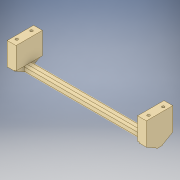
# Autodesk Inventor part: Handle
Saved by Autodesk Inventor 2019 (Build 230136000, 136)
## iProperties
Created: 2020-03-14
Part Number: Handle
Material: Generic
Document SubType Name: Modeling
Designer: james
Density: 1 g/cm^3
Appearance: Beige
Author: james
Autodesk Inventor part; units mm, degrees
ref_plane "YZ Plane" through (0, 0, 0) normal (1, 0, 0) x (0, 1, 0)
ref_plane "XZ Plane" through (0, 0, 0) normal (0, 1, 0) x (-1, 0, 0)
ref_plane "XY Plane" through (0, 0, 0) normal (0, 0, 1) x (1, 0, 0)
sketch "Sketch1" plane through (0, 0, 0) normal (1, 0, 0) x (0, 1, 0)
  line L0 (7.7549, 10.0308) -> (1.4049, 10.0308)
  line L1 (-1.7701, 6.8558) -> (-1.7701, 0.5058)
  line L2 (1.4049, -2.6692) -> (7.7549, -2.6692)
  line L3 (10.9299, 0.5058) -> (10.9299, 6.8558)
  arc A0 (10.9299, 6.8558) -> (7.7549, 10.0308) centre (7.7549, 6.8558) ccw
  arc A1 (7.7549, -2.6692) -> (10.9299, 0.5058) centre (7.7549, 0.5058) ccw
  arc A2 (-1.7701, 0.5058) -> (1.4049, -2.6692) centre (1.4049, 0.5058) ccw
  arc A3 (1.4049, 10.0308) -> (-1.7701, 6.8558) centre (1.4049, 6.8558) ccw
  point P0 (0, 0)
  point P1 (10.9299, 10.0308)
  point P2 (-1.7701, -2.6692)
  point P3 (-1.7701, 10.0308)
  dimension "d0" = 12.7
  dimension "d1" = 12.7
  dimension "d2" = 3.175
  constraints: 8 end point, 8 point on circle, 8 tangent, 6 point on line, 4 centre point, 3 equal radius, 2 parallel, 1 horizontal, 1 perpendicular
  measures "d0" distance of point (-1.77, 10.031) point (-1.77, -2.669)
  measures "d1" distance of point (10.93, 10.031) point (-1.77, 10.031)
  measures "d2" radius of A0
extrude "Extrusion1" add sketch "Sketch1" along normal blind 241.3
sketch "Sketch2" plane through (0, 10.9299, 6.8558) normal (0, 1, 0) x (1, 0, 0)
  line L0 (0, -22.225) -> (15.24, -22.225)
  line L1 (15.24, -22.225) -> (15.24, 28.575)
  line L2 (15.24, 28.575) -> (0, 28.575)
  line L3 (0, 28.575) -> (0, -22.225)
  line L4 (0, -3.175) -> (241.3, -3.175) projected
  line L5 (0, 9.525) -> (241.3, 9.525) projected
  line L6 (226.06, -22.225) -> (241.3, -22.225)
  line L7 (241.3, -22.225) -> (241.3, 28.575)
  line L8 (241.3, 28.575) -> (226.06, 28.575)
  line L9 (226.06, 28.575) -> (226.06, -22.225)
  line L10 (241.3, 6.35) -> (241.3, 0) projected
  point P0 (0, 6.8558)
  dimension "d5" = 19.05
  dimension "d6" = 19.05
  dimension "d7" = 15.24
  dimension "d8" = 0
  dimension "d9" = 19.05
  dimension "d10" = 19.05
  dimension "d11" = 15.24
  constraints: 16 end point, 4 parallel, 2 horizontal, 2 perpendicular
  measures "d5" distance between parallel lines of L4 L0
  measures "d6" distance between parallel lines of L5 L2
  measures "d7" distance between parallel lines of L1 L3
  measures "d8" distance between parallel lines of L10 L7
  measures "d9" distance between parallel lines of L5 L8
  measures "d10" distance between parallel lines of L4 L6
  measures "d11" distance between parallel lines of L7 L9
extrude "Extrusion2" add sketch "Sketch2" along normal blind 38.1 contours L3 L4 L1 L0 | L3 L5 L1 L4 | L3 L2 L1 L5 | L9 L5 L7 L4 | L4 L7 L6 L9 | L9 L8 L7 L5
sketch "Sketch4" plane through (241.3, 0, 0) normal (1, 0, 0) x (0, 0, -1)
  line L0 (-29.0808, 10.9299) -> (-6.8558, 10.9299) projected
  line L1 (-0.5058, 10.9299) -> (21.7192, 10.9299) projected
  line L2 (-6.8558, -1.7701) -> (-0.5058, -1.7701) projected
  line L3 (-6.8558, -1.7701) -> (-29.0808, 10.9299)
  line L4 (-6.8558, -1.7701) -> (-0.5058, -1.7701) projected
  line L5 (-0.5058, -1.7701) -> (21.7192, 10.9299)
  line L6 (-0.5058, -1.7701) -> (-6.8558, -1.7701)
  line L7 (-6.8558, 10.9299) -> (-29.0808, 10.9299) projected
  line L8 (21.7192, 10.9299) -> (-29.0808, 10.9299)
  point P0 (0, 0)
  constraints: 8 end point, 2 collinear
extrude "Extrusion3" add sketch "Sketch4" against normal blind 12.7
sketch "Sketch3" plane through (0, 49.0299, 6.8558) normal (0, 1, 0) x (1, 0, 0)
  line L0 (0, -22.225) -> (15.24, -22.225) projected
  line L1 (0, 28.575) -> (0, -22.225) projected
  line L2 (241.3, -22.225) -> (241.3, 28.575) projected
  line L3 (241.3, 28.575) -> (226.06, 28.575) projected
  line L4 (226.06, -22.225) -> (241.3, -22.225) projected
  point P0 (0, 6.8558)
  point P1 (6.35, -9.525)
  point P2 (6.35, 15.875)
  point P3 (234.95, -9.525)
  point P4 (234.95, 15.875)
  dimension "d14" = 25.4
  dimension "d15" = 12.7
  dimension "d16" = 0
  dimension "d17" = 6.35
  dimension "d18" = 0
  dimension "d19" = 6.35
  dimension "d20" = 12.7
  dimension "d21" = 12.7
  measures "d14" distance of point (6.35, -9.525) point (6.35, 15.875)
  measures "d15" distance from line of L0 point (6.35, -9.525)
  measures "d16" horizontal distance of point (6.35, 15.875) point (6.35, -9.525)
  measures "d17" distance from line of L1 point (6.35, 15.875)
  measures "d18" horizontal distance of point (234.95, 15.875) point (234.95, -9.525)
  measures "d19" distance from line of L2 point (234.95, 15.875)
  measures "d20" distance from line of L3 point (234.95, 15.875)
  measures "d21" distance from line of L4 point (234.95, -9.525)
hole "Hole1" at (6.35, 49.0299, 16.3808) at (6.35, 49.0299, -9.0192) at (234.95, 49.0299, 16.3808) at (234.95, 49.0299, -9.0192) direction (0, -1, 0) diameter 4.4958 depth 25.4 tip angle 118 clearance for "Flat Head Machine Screw (82)" size "#8" standard "Ansi Unified Screw Threads"
sketch "Sketch5" plane through (0, 0, 0) normal (-1, 0, 0) x (0, 0, 1)
  line L0 (6.8558, -1.7701) -> (0.5058, -1.7701) projected
  line L1 (6.8558, 10.9299) -> (29.0808, 10.9299) projected
  line L2 (-21.7192, 10.9299) -> (0.5058, 10.9299) projected
  line L3 (-21.7192, 10.9299) -> (-2.2296, -0.2071) projected
  line L4 (29.0808, 10.9299) -> (-21.7192, 10.9299)
  line L5 (-21.7192, 10.9299) -> (0.5058, -1.7701)
  line L6 (6.8558, -1.7701) -> (0.5058, -1.7701) projected
  line L7 (29.0808, 10.9299) -> (29.0808, 49.0299) projected
  line L8 (6.8558, -1.7701) -> (29.0808, 10.9299)
  point P0 (0, 0)
  constraints: 6 end point, 1 collinear, 1 horizontal
extrude "Extrusion4" add sketch "Sketch5" against normal blind 12.7
sketch "Sketch6" plane through (0, 49.0299, 6.8558) normal (0, 1, 0) x (1, 0, 0)
  circle A0 centre (6.35, -9.525) radius 2.2479 projected
  circle A1 centre (6.35, 15.875) radius 2.2479 projected
  circle A2 centre (234.95, -9.525) radius 2.2479 projected
  circle A3 centre (234.95, 15.875) radius 2.2479 projected
  circle A4 centre (234.95, -9.525) radius 2.2479 projected
  point P0 (0, 6.8558)
  constraints: 4 coincident
hole "Hole2" at (234.95, 49.0299, 16.3808) at (234.95, 49.0299, -9.0192) at (6.35, 49.0299, -9.0192) at (6.35, 49.0299, 16.3808) direction (0, -1, 0) diameter 4.4958 end through all clearance for "Flat Head Machine Screw (82)" size "#8" standard "Ansi Unified Screw Threads"
sketch "Sketch7" plane through (0, -1.7701, 0.5058) normal (0, -1, 0) x (1, 0, 0)
  circle A0 centre (6.35, -9.525) radius 2.2479 projected
  circle A1 centre (6.35, 15.875) radius 2.2479 projected
  circle A2 centre (234.95, 15.875) radius 2.2479 projected
  circle A3 centre (234.95, -9.525) radius 2.2479 projected
  circle A4 centre (234.95, -9.525) radius 5.08
  circle A5 centre (234.95, 15.875) radius 5.08
  circle A6 centre (6.35, -9.525) radius 5.08
  circle A7 centre (6.35, 15.875) radius 5.08
  point P0 (0, -0.5058)
  dimension "d40" = 10.16
  dimension "d41" = 10.16
  dimension "d42" = 10.16
  dimension "d43" = 10.16
  constraints: 4 centre point, 4 coincident
  measures "d40" diameter of A4
  measures "d41" diameter of A5
  measures "d42" diameter of A6
  measures "d43" diameter of A7
extrude "Extrusion5" cut sketch "Sketch7" against normal blind 12.7
sketch "Sketch8" plane through (0, 49.0299, 6.8558) normal (0, 1, 0) x (1, 0, 0)
  line L0 (261.8512, -57.5381) -> (-18.787, -57.5381)
  line L1 (-18.787, -57.5381) -> (-18.787, -19.685)
  line L2 (-18.787, -19.685) -> (261.8512, -19.685)
  line L3 (261.8512, -19.685) -> (261.8512, -57.5381)
  line L4 (261.8512, 26.035) -> (-15.1591, 26.035)
  line L5 (-15.1591, 26.035) -> (-15.1591, 48.4462)
  line L6 (-15.1591, 48.4462) -> (261.8512, 48.4462)
  line L7 (261.8512, 48.4462) -> (261.8512, 26.035)
  line L8 (226.06, -22.225) -> (241.3, -22.225) projected
  line L9 (241.3, 28.575) -> (226.06, 28.575) projected
  point P0 (0, 6.8558)
  dimension "d46" = 2.54
  dimension "d47" = 2.54
  constraints: 16 end point, 4 parallel, 2 horizontal, 2 perpendicular, 1 point on line
  measures "d46" distance between parallel lines of L8 L2
  measures "d47" distance between parallel lines of L9 L4
extrude "Extrusion6" cut sketch "Sketch8" against normal blind 71.4375
body "Solid1"
